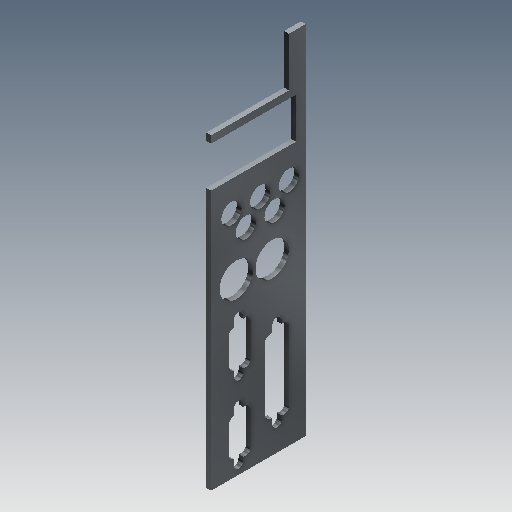
# Autodesk Inventor part: config - casing - module protector
Saved by Autodesk Inventor 2019.1 (Build 231200000, 200)
## iProperties
Company: Autodesk Asia Pte. Ltd.
Created: 2005-12-16
Part Number: config - casing - module protector
Document SubType Name: Modeling
Designer: Simon.Ng@autodesk.com
Density: 1 g/cm^3
Material: Generic
Description: Module Protector
Appearance: Zinc
Mass: 6.64671 g
Surface Area: 84.1526 cm^2
Volume: 6.64671 cm^3
Title: Purchased Part
Author: Simon.Ng@autodesk.com
Autodesk Inventor part; units mm, degrees
ref_plane "YZ Plane" through (0, 0, 0) normal (1, 0, 0) x (0, 1, 0)
ref_plane "XZ Plane" through (0, 0, 0) normal (0, 1, 0) x (-1, 0, 0)
ref_plane "XY Plane" through (0, 0, 0) normal (0, 0, 1) x (1, 0, 0)
sketch "Sketch2" plane through (0, 0, 0) normal (1, 0, 0) x (0, 1, 0)
  line L0 (-2.5, 55.99) -> (-2.5, 18.99)
  line L1 (-2.5, 18.99) -> (-150.5, 18.99)
  line L2 (-150.5, 18.99) -> (-150.5, 55.99)
  line L3 (-150.5, 55.99) -> (-2.5, 55.99)
  line L4 (87, 57.49) -> (-160.5, 57.49)
  line L5 (-151, 57.49) -> (-2, 57.49)
  line L6 (-2, 57.49) -> (-2, 17.99)
  line L7 (-2, 17.99) -> (-151, 17.99)
  line L8 (-151, 17.99) -> (-151, 57.49)
  dimension "d1" = 1.5
  dimension "d2" = 0.5
  dimension "d3" = 0.5
  dimension "d4" = 1
  constraints: 18 end point, 2 parallel, 1 horizontal, 1 perpendicular, 1 point on line
  measures "d1" distance between parallel lines of L4 L3
  measures "d2" distance between parallel lines of L0 L6
  measures "d3" distance between parallel lines of L2 L8
  measures "d4" distance between parallel lines of L7 L1
extrude "Extrusion1" add sketch "Sketch2" along normal blind 2 contours L0 L1 L2 L3 | L6 L7 L8 L4
sketch "Sketch3" plane through (0, 0, 0) normal (-1, 0, 0) x (0, -1, 0)
  arc A0 (111.6743, 41.99) -> (112.6358, 43.2647) centre (111.6743, 42.99) ccw
  line L0 (111.2072, 48.2647) -> (112.6358, 43.2647)
  arc A1 (111.2072, 48.2647) -> (110.2457, 48.99) centre (110.2457, 47.99) ccw
  line L1 (98.7543, 48.99) -> (110.2457, 48.99)
  arc A2 (98.7543, 48.99) -> (97.7928, 48.2647) centre (98.7543, 47.99) ccw
  line L2 (96.3642, 43.2647) -> (97.7928, 48.2647)
  arc A3 (96.3642, 43.2647) -> (97.3257, 41.99) centre (97.3257, 42.99) ccw
  line L3 (111.6743, 41.99) -> (97.3257, 41.99)
  circle A4 centre (114.8571, 45.99) radius 0.7915
  circle A5 centre (94.1429, 45.99) radius 0.7915
  line L4 (143.6743, 41.99) -> (129.3257, 41.99)
  arc A6 (128.3642, 43.2647) -> (129.3257, 41.99) centre (129.3257, 42.99) ccw
  line L5 (128.3642, 43.2647) -> (129.7928, 48.2647)
  arc A7 (130.7543, 48.99) -> (129.7928, 48.2647) centre (130.7543, 47.99) ccw
  line L6 (130.7543, 48.99) -> (142.2457, 48.99)
  arc A8 (143.2072, 48.2647) -> (142.2457, 48.99) centre (142.2457, 47.99) ccw
  line L7 (143.2072, 48.2647) -> (144.6358, 43.2647)
  arc A9 (143.6743, 41.99) -> (144.6358, 43.2647) centre (143.6743, 42.99) ccw
  circle A10 centre (146.8571, 45.99) radius 0.7915
  circle A11 centre (126.1429, 45.99) radius 0.7915
  line L8 (108.7808, 33.99) -> (135.2192, 33.99)
  arc A12 (108.7808, 33.99) -> (107.8106, 33.2325) centre (108.7808, 32.99) ccw
  line L9 (106.3106, 27.2325) -> (107.8106, 33.2325)
  arc A13 (106.3106, 27.2325) -> (107.2808, 25.99) centre (107.2808, 26.99) ccw
  line L10 (136.7192, 25.99) -> (107.2808, 25.99)
  arc A14 (136.7192, 25.99) -> (137.6894, 27.2325) centre (136.7192, 26.99) ccw
  line L11 (136.1894, 33.2325) -> (137.6894, 27.2325)
  arc A15 (136.1894, 33.2325) -> (135.2192, 33.99) centre (135.2192, 32.99) ccw
  circle A16 centre (140, 29.99) radius 0.7915
  circle A17 centre (104, 29.99) radius 0.7915
  arc A18 (95.4027, 43.5394) -> (97.3257, 40.99) centre (97.3257, 42.99) ccw
  line L12 (95.4027, 43.5394) -> (96.8313, 48.5394)
  arc A19 (98.7543, 49.99) -> (96.8313, 48.5394) centre (98.7543, 47.99) ccw
  line L13 (98.7543, 49.99) -> (110.2457, 49.99)
  arc A20 (112.1687, 48.5394) -> (110.2457, 49.99) centre (110.2457, 47.99) ccw
  line L14 (112.1687, 48.5394) -> (113.5973, 43.5394)
  arc A21 (111.6743, 40.99) -> (113.5973, 43.5394) centre (111.6743, 42.99) ccw
  line L15 (111.6743, 40.99) -> (97.3257, 40.99)
  circle A22 centre (94.1429, 45.99) radius 2
  line L16 (94.1429, 47.99) -> (96.6743, 47.99)
  line L17 (94.1429, 43.99) -> (95.5314, 43.99)
  circle A23 centre (114.8571, 45.99) radius 2
  line L18 (114.8571, 47.99) -> (112.3257, 47.99)
  line L19 (114.8571, 43.99) -> (113.4686, 43.99)
  circle A24 centre (126.1429, 45.99) radius 2
  circle A25 centre (146.8571, 45.99) radius 2
  circle A26 centre (140, 29.99) radius 2
  circle A27 centre (104, 29.99) radius 2
  line L20 (142.2457, 49.99) -> (130.7543, 49.99)
  arc A28 (130.7543, 49.99) -> (128.8313, 48.5394) centre (130.7543, 47.99) ccw
  line L21 (128.8313, 48.5394) -> (127.4027, 43.5394)
  arc A29 (127.4027, 43.5394) -> (129.3257, 40.99) centre (129.3257, 42.99) ccw
  line L22 (129.3257, 40.99) -> (143.6743, 40.99)
  arc A30 (143.6743, 40.99) -> (145.5973, 43.5394) centre (143.6743, 42.99) ccw
  line L23 (145.5973, 43.5394) -> (144.1687, 48.5394)
  arc A31 (144.1687, 48.5394) -> (142.2457, 49.99) centre (142.2457, 47.99) ccw
  line L24 (126.1429, 47.99) -> (128.6743, 47.99)
  line L25 (126.1429, 43.99) -> (127.5314, 43.99)
  line L26 (146.8571, 47.99) -> (144.3257, 47.99)
  line L27 (146.8571, 43.99) -> (145.4686, 43.99)
  line L28 (135.2192, 34.99) -> (108.7808, 34.99)
  arc A32 (108.7808, 34.99) -> (106.8405, 33.4751) centre (108.7808, 32.99) ccw
  line L29 (106.8405, 33.4751) -> (105.3405, 27.4751)
  arc A33 (105.3405, 27.4751) -> (107.2808, 24.99) centre (107.2808, 26.99) ccw
  line L30 (107.2808, 24.99) -> (136.7192, 24.99)
  arc A34 (136.7192, 24.99) -> (138.6595, 27.4751) centre (136.7192, 26.99) ccw
  line L31 (138.6595, 27.4751) -> (137.1595, 33.4751)
  arc A35 (137.1595, 33.4751) -> (135.2192, 34.99) centre (135.2192, 32.99) ccw
  line L32 (104, 31.99) -> (106.4692, 31.99)
  line L33 (104, 27.99) -> (105.4692, 27.99)
  line L34 (140, 31.99) -> (137.5308, 31.99)
  line L35 (140, 27.99) -> (138.5308, 27.99)
  dimension "d7" = 1
  dimension "d8" = 4
  dimension "d9" = 1
  dimension "d10" = 1
  constraints: 72 end point, 60 point on circle, 36 centre point, 12 parallel, 12 point on line, 12 tangent, 6 coincident, 6 horizontal, 5 equal radius, 87 other
  measures "d7" distance between parallel lines of L1 L13
  measures "d8" diameter of A22
  measures "d9" distance between parallel lines of L6 L20
  measures "d10" distance between parallel lines of L8 L28
extrude "Extrusion2" cut sketch "Sketch3" against normal through all contours L3 A3 L2 A2 L1 A1 L0 A0 | A4 | A5 | L4 A6 L5 A7 L6 A8 L7 A9 | A10 | A11 | L8 A15 L11 A14 L10 A13 L9 A12 | A16 | A17 | L12 A22 A19 L13 A20 L14 A23 A21 L15 A18 | L17 A22 L12 | A22 L12 | L12 A22 | A22 L16 L12 | L14 A23 L19 | A23 L14 | L14 A23 | L14 L18 A23 | A24 L21 | L24 L21 A24 | A24 L21 L25 | L21 A28 L20 A31 L23 A25 A30 L22 A29 A24 | A24 L21 | L26 A25 L23 | L23 A25 L27 | L23 A25 | A25 L23 | A26 L31 | A26 L31 L34 | L35 L31 A26 | L31 A26 | A26 L31 A34 L30 A33 L29 A27 A32 L28 A35 | L29 A27 L32 | L33 A27 L29 | L29 A27 | A27 L29
sketch "Sketch4" plane through (0, 0, 0) normal (-1, 0, 0) x (0, -1, 0)
  circle A0 centre (55, 48.99) radius 3.5
  circle A1 centre (63, 42.99) radius 3.5
  circle A2 centre (55, 36.99) radius 3.5
  circle A3 centre (63, 30.99) radius 3.5
  circle A4 centre (55, 24.99) radius 3.5
  circle A5 centre (80, 46.99) radius 6
  circle A6 centre (80, 31.99) radius 6
  circle A7 centre (55, 48.99) radius 4.25
  circle A8 centre (63, 42.99) radius 4.25
  circle A9 centre (55, 36.99) radius 4.25
  circle A10 centre (55, 24.99) radius 4.25
  circle A11 centre (63, 30.99) radius 4.25
  circle A12 centre (80, 31.99) radius 7
  circle A13 centre (80, 46.99) radius 7
  dimension "d13" = 8.5
  dimension "d14" = 14
  constraints: 14 centre point, 7 coincident, 5 equal radius, 14 other
  measures "d13" diameter of A7
  measures "d14" diameter of A13
extrude "Extrusion3" cut sketch "Sketch4" against normal through all contours A0 | A1 | A2 | A3 | A4 | A5 | A6 | A7 | A8 | A9 | A10 | A11 | A12 | A13
sketch "Sketch5" plane through (0, 0, 0) normal (-1, 0, 0) x (0, -1, 0)
  line L0 (2, 57.49) -> (151, 57.49) projected
  line L1 (2, 17.99) -> (2, 57.49) projected
  line L2 (2, 24.99) -> (22.5, 24.99)
  line L3 (22.5, 24.99) -> (22.5, 57.49)
  line L4 (22.5, 57.49) -> (2, 57.49)
  line L5 (2, 57.49) -> (2, 24.99)
  line L6 (25.5, 21.99) -> (42.5, 21.99)
  line L7 (42.5, 21.99) -> (42.5, 57.49)
  line L8 (42.5, 57.49) -> (25.5, 57.49)
  line L9 (25.5, 57.49) -> (25.5, 21.99)
  line L10 (151, 17.99) -> (2, 17.99) projected
  dimension "d24" = 4
  dimension "d25" = 7
  dimension "d26" = 20.5
  dimension "d27" = 3
  dimension "d28" = 17
  constraints: 16 end point, 4 parallel, 3 point on line, 2 horizontal, 2 perpendicular
  measures "d24" distance between parallel lines of L10 L6
  measures "d25" distance between parallel lines of L10 L2
  measures "d26" distance of L2.start L2.end
  measures "d27" distance between parallel lines of L9 L3
  measures "d28" distance between parallel lines of L7 L9
extrude "Extrusion4" cut sketch "Sketch5" against normal through all
equation "\"d9\" = d7"
equation "\"d10\" = d7"
body "Solid1"
